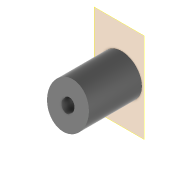
# Autodesk Inventor part: spacer electronica
Saved by Autodesk Inventor 2020.3 (Build 243373000, 373)
## iProperties
Created: 2020-10-19
Part Number: spacer electronica
Material: ABS Plastic
Document SubType Name: Modeling
Designer: Svend
Density: 1.06 g/cm^3
Appearance: Smooth - White
Author: Svend
Autodesk Inventor part; units mm, degrees
ref_plane "YZ Plane" through (0, 0, 0) normal (1, 0, 0) x (0, 1, 0)
ref_plane "XZ Plane" through (0, 0, 0) normal (0, 1, 0) x (-1, 0, 0)
ref_plane "Work Plane1" through (0, 0, 0) normal (0, 0, 1) x (1, 0, 0)
sketch "Sketch1" plane through (0, 0, 0) normal (0, 0, 1) x (1, 0, 0)
  circle A0 centre (-17.9615, 30) radius 10 projected
  circle A1 centre (-17.9615, 30) radius 10 projected
  line L0 (-25.9615, 43.8564) -> (-5, 55.9585) projected
  arc A2 (-25.9615, 43.8564) -> (-25.9615, 16.1436) centre (-17.9615, 30) ccw projected
  line L1 (-5, 4.0415) -> (-25.9615, 16.1436) projected
  line L2 (-5, 55.9585) -> (-5, 4.0415) projected
  circle A3 centre (-392.0385, 30) radius 10 projected
  line L3 (-384.0385, 43.8564) -> (-405, 55.9585) projected
  line L4 (-405, 55.9585) -> (-405, 4.0415) projected
  line L5 (-405, 4.0415) -> (-384.0385, 16.1436) projected
  arc A4 (-384.0385, 16.1436) -> (-384.0385, 43.8564) centre (-392.0385, 30) ccw projected
  circle A5 centre (-17.9615, 30) radius 12.9615
  point P0 (0, 0)
  constraints: 1 centre point, 1 coincident, 1 tangent
ref_plane "Work Plane2" through (-405, -106.0272, 65.4176) normal (0, -0.225, -0.9744) x (0, 0.9744, -0.225)
extrude "Extrusion1" add sketch "Sketch1" along normal up to surface contours A0 | A5 surface through (-405, -106.0272, 65.4176) normal (0, -0.225, -0.9744)
sketch "Sketch2" plane through (-17.9615, 30, 0) normal (0, 0, -1) x (-1, 0, 0)
  circle A0 centre (0, 0) radius 12.9615 projected
  point P0 (-17.9615, -30)
  constraints: 1 coincident
hole "Hole1" at (-17.9615, 30, 0) direction (0, 0, 1) diameter 8 depth 45.1 tip angle 90
body "Solid1"
